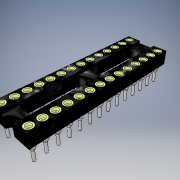
# Autodesk Inventor part: DIL28-Socket
Saved by Autodesk Inventor 2018 (Build 220112000, 112)
## iProperties
Created: 2020-04-18
Part Number: DIL28-Socket
Material: Všeobecné
Document SubType Name: Modeling
Designer: Jozko Mrkvicka
Density: 1 g/cm^3
Appearance: Výchozí
Author: Jozko Mrkvicka
Autodesk Inventor part; units mm, degrees
ref_plane "YZ Plane" through (0, 0, 0) normal (1, 0, 0) x (0, 1, 0)
ref_plane "XZ Plane" through (0, 0, 0) normal (0, 1, 0) x (-1, 0, 0)
ref_plane "XY Plane" through (0, 0, 0) normal (0, 0, 1) x (1, 0, 0)
sketch "Náčrt1" plane through (0, 0, 0) normal (0, 1, 0) x (-1, 0, 0)
  line L0 (10.16, 0) -> (10.16, -35.56)
  line L1 (10.16, -35.56) -> (0, -35.56)
  line L2 (0, -35.56) -> (0, 0)
  line L3 (0, 0) -> (3.175, 0)
  line L4 (3.175, -35.56) -> (0, -35.56)
  line L5 (0, -35.56) -> (0, 0)
  line L6 (10.16, 0) -> (6.985, 0)
  line L7 (6.985, -35.56) -> (10.16, -35.56)
  line L8 (10.16, -35.56) -> (10.16, 0)
  line L9 (3.81, -3.175) -> (6.35, -3.175)
  line L10 (6.985, -35.56) -> (3.175, -35.56)
  line L11 (3.81, -32.385) -> (6.35, -32.385)
  line L12 (3.81, -16.1925) -> (6.35, -16.1925)
  line L13 (6.35, -19.3675) -> (3.81, -19.3675)
  line L14 (6.985, -3.81) -> (6.985, -15.5575)
  line L15 (6.985, -20.0025) -> (6.985, -31.75)
  line L16 (3.175, -3.81) -> (3.175, -15.5575)
  line L17 (3.175, -20.0025) -> (3.175, -31.75)
  arc A0 (3.81, 0) -> (6.35, 0) centre (5.08, 0) ccw
  line L18 (0, 0) -> (3.81, 0)
  line L19 (6.35, 0) -> (10.16, 0)
  line L20 (6.985, 0) -> (6.35, 0)
  line L21 (3.81, 0) -> (3.175, 0)
  arc A1 (6.985, -3.81) -> (6.35, -3.175) centre (6.35, -3.81) ccw
  arc A2 (3.81, -3.175) -> (3.175, -3.81) centre (3.81, -3.81) ccw
  arc A3 (3.175, -15.5575) -> (3.81, -16.1925) centre (3.81, -15.5575) ccw
  arc A4 (6.35, -16.1925) -> (6.985, -15.5575) centre (6.35, -15.5575) ccw
  arc A5 (6.985, -20.0025) -> (6.35, -19.3675) centre (6.35, -20.0025) ccw
  arc A6 (3.81, -19.3675) -> (3.175, -20.0025) centre (3.81, -20.0025) ccw
  arc A7 (6.35, -32.385) -> (6.985, -31.75) centre (6.35, -31.75) ccw
  arc A8 (3.175, -31.75) -> (3.81, -32.385) centre (3.81, -31.75) ccw
  dimension "d0" = 10.16
  dimension "d1" = 35.56
  dimension "d6" = 2.54
  dimension "d7" = 0.635
  constraints: 44 end point, 18 point on circle, 16 tangent, 13 parallel, 9 centre point, 8 horizontal, 7 equal radius, 6 perpendicular, 2 point on line
  measures "d0" distance of L0.end L1.end
  measures "d1" distance of L0.start L0.end
  measures "d6" diameter of A0
  measures "d7" radius of A1
extrude "Vysunutí1" add sketch "Náčrt1" along normal blind 3.175
sketch "Náčrt2" plane through (0, 3.175, 0) normal (0, 1, 0) x (1, 0, 0)
  line L0 (-6.985, 3.81) -> (-6.985, 15.5575) projected
  line L1 (-6.985, 3.81) -> (-3.1004, 3.81)
  line L2 (0, 35.56) -> (-10.16, 35.56) projected
  line L3 (-6.985, 3.81) -> (-3.175, 3.81)
  line L4 (-3.175, 3.81) -> (-3.175, 35.56)
  line L5 (-3.175, 35.56) -> (-6.985, 35.56)
  line L6 (-6.985, 35.56) -> (-6.985, 3.81)
  line L7 (-3.81, 0) -> (0, 0) projected
  line L8 (-6.985, 3.81) -> (-3.175, 3.81)
  line L9 (-3.175, 3.81) -> (-3.175, 0)
  line L10 (-3.175, 0) -> (-6.985, 0)
  line L11 (-6.985, 0) -> (-6.985, 3.81)
  constraints: 18 end point, 4 parallel, 3 horizontal, 2 perpendicular, 2 point on line
extrude "Vysunutí2" cut sketch "Náčrt2" against normal blind 0.635
sketch "Náčrt3" plane through (0, 0, 0) normal (0, -1, 0) x (1, 0, 0)
  circle A0 centre (-1.27, -1.27) radius 0.635
  circle A1 centre (-1.27, -3.81) radius 0.635
  circle A2 centre (-1.27, -6.35) radius 0.635
  circle A3 centre (-1.27, -8.89) radius 0.635
  circle A4 centre (-1.27, -11.43) radius 0.635
  circle A5 centre (-1.27, -13.97) radius 0.635
  circle A6 centre (-1.27, -16.51) radius 0.635
  circle A7 centre (-1.27, -19.05) radius 0.635
  circle A8 centre (-1.27, -21.59) radius 0.635
  circle A9 centre (-8.89, -1.27) radius 0.635
  circle A10 centre (-8.89, -3.81) radius 0.635
  circle A11 centre (-8.89, -6.35) radius 0.635
  circle A12 centre (-8.89, -8.89) radius 0.635
  circle A13 centre (-8.89, -34.29) radius 0.635
  circle A14 centre (-8.89, -31.75) radius 0.635
  circle A15 centre (-8.89, -29.21) radius 0.635
  circle A16 centre (-8.89, -26.67) radius 0.635
  circle A17 centre (-8.89, -24.13) radius 0.635
  circle A18 centre (-8.89, -21.59) radius 0.635
  circle A19 centre (-8.89, -19.05) radius 0.635
  circle A20 centre (-8.89, -16.51) radius 0.635
  circle A21 centre (-8.89, -13.97) radius 0.635
  circle A22 centre (-8.89, -11.43) radius 0.635
  circle A23 centre (-1.27, -34.29) radius 0.635
  circle A24 centre (-1.27, -31.75) radius 0.635
  circle A25 centre (-1.27, -29.21) radius 0.635
  circle A26 centre (-1.27, -26.67) radius 0.635
  circle A27 centre (-1.27, -24.13) radius 0.635
  point P0 (0, 0)
  point P1 (-8.89, -1.27)
  point P2 (-8.89, -3.81)
  point P3 (-8.89, -6.35)
  point P4 (-8.89, -8.89)
  point P5 (-8.89, -11.43)
  point P6 (-8.89, -13.97)
  point P7 (-8.89, -16.51)
  point P8 (-8.89, -19.05)
  point P9 (-8.89, -21.59)
  point P10 (-8.89, -24.13)
  point P11 (-8.89, -26.67)
  point P12 (-8.89, -29.21)
  point P13 (-8.89, -31.75)
  point P14 (-8.89, -34.29)
  point P15 (-1.27, -1.27)
  point P16 (-1.27, -3.81)
  point P17 (-1.27, -11.43)
  point P18 (-1.27, -13.97)
  point P19 (-1.27, -16.51)
  point P20 (-1.27, -19.05)
  point P21 (-1.27, -21.59)
  point P22 (-1.27, -24.13)
  point P23 (-1.27, -26.67)
  point P24 (-1.27, -29.21)
  point P25 (-1.27, -31.75)
  point P26 (-1.27, -34.29)
  constraints: 28 centre point, 1 coincident
extrude "Vysunutí3" add sketch "Náčrt3" along normal blind 1.905
chamfer "Zkosení1" distance 0.3175 distance2 0.635 1 edges at (-1.905, -1.905, -1.27) measured on face at (-1.0935, -1.905, -1.2787)
chamfer "Zkosení2" distance 0.3175 distance2 0.635 1 edges at (-1.905, -1.905, -13.97) measured on face at (-1.4636, -1.905, -14.0177)
chamfer "Zkosení3" distance 0.3175 distance2 0.635 1 edges at (-1.905, -1.905, -3.81) measured on face at (-1.2445, -1.905, -4.0201)
chamfer "Zkosení4" distance 0.3175 distance2 0.635 1 edges at (-9.525, -1.905, -1.27) measured on face at (-8.6964, -1.905, -1.419)
chamfer "Zkosení5" distance 0.3175 distance2 0.635 1 edges at (-9.525, -1.905, -3.81) measured on face at (-8.6964, -1.905, -3.959)
chamfer "Zkosení6" distance 0.3175 distance2 0.635 1 edges at (-9.525, -1.905, -6.35) measured on face at (-8.6964, -1.905, -6.499)
chamfer "Zkosení7" distance 0.3175 distance2 0.635 1 edges at (-9.525, -1.905, -8.89) measured on face at (-8.6783, -1.905, -9.0867)
chamfer "Zkosení8" distance 0.3175 distance2 0.635 1 edges at (-9.525, -1.905, -11.43) measured on face at (-8.6783, -1.905, -11.6267)
chamfer "Zkosení9" distance 0.3175 distance2 0.635 1 edges at (-9.525, -1.905, -13.97) measured on face at (-8.6783, -1.905, -14.1667)
chamfer "Zkosení10" distance 0.3175 distance2 0.635 1 edges at (-1.905, -1.905, -6.35) measured on face at (-1.0645, -1.905, -6.4007)
chamfer "Zkosení11" distance 0.3175 distance2 0.635 1 edges at (-1.905, -1.905, -8.89) measured on face at (-1.4636, -1.905, -8.9377)
chamfer "Zkosení12" distance 0.3175 distance2 0.635 1 edges at (-1.905, -1.905, -11.43) measured on face at (-1.4636, -1.905, -11.4777)
chamfer "Zkosení13" distance 0.3175 distance2 0.635 1 edges at (-1.905, -1.905, -16.51) measured on face at (-1.0826, -1.905, -16.5129)
chamfer "Zkosení14" distance 0.3175 distance2 0.635 1 edges at (-9.525, -1.905, -16.51) measured on face at (-8.7026, -1.905, -16.4116)
chamfer "Zkosení15" distance 0.3175 distance2 0.635 1 edges at (-9.525, -1.905, -19.05) measured on face at (-8.7026, -1.905, -18.9516)
chamfer "Zkosení16" distance 0.3175 distance2 0.635 1 edges at (-1.905, -1.905, -19.05) measured on face at (-1.0826, -1.905, -19.0529)
chamfer "Zkosení17" distance 0.3175 distance2 0.635 1 edges at (-1.905, -1.905, -21.59) measured on face at (-1.0826, -1.905, -21.5929)
chamfer "Zkosení18" distance 0.3175 distance2 0.635 1 edges at (-1.905, -1.905, -24.13) measured on face at (-1.0826, -1.905, -24.1329)
chamfer "Zkosení19" distance 0.3175 distance2 0.635 1 edges at (-1.905, -1.905, -26.67) measured on face at (-1.0826, -1.905, -26.6729)
chamfer "Zkosení20" distance 0.3175 distance2 0.635 1 edges at (-1.905, -1.905, -29.21) measured on face at (-1.0826, -1.905, -29.2129)
chamfer "Zkosení21" distance 0.3175 distance2 0.635 1 edges at (-1.905, -1.905, -31.75) measured on face at (-1.2445, -1.905, -31.9357)
chamfer "Zkosení22" distance 0.3175 distance2 0.635 1 edges at (-1.905, -1.905, -34.29) measured on face at (-1.3451, -1.905, -34.0921)
chamfer "Zkosení23" distance 0.3175 distance2 0.635 1 edges at (-9.525, -1.905, -34.29) measured on face at (-9.2437, -1.905, -34.1259)
chamfer "Zkosení24" distance 0.3175 distance2 0.635 1 edges at (-9.525, -1.905, -31.75) measured on face at (-8.8645, -1.905, -31.9357)
chamfer "Zkosení25" distance 0.3175 distance2 0.635 1 edges at (-9.525, -1.905, -29.21) measured on face at (-8.7026, -1.905, -29.1116)
chamfer "Zkosení26" distance 0.3175 distance2 0.635 1 edges at (-9.525, -1.905, -26.67) measured on face at (-8.7026, -1.905, -26.5716)
chamfer "Zkosení27" distance 0.3175 distance2 0.635 1 edges at (-9.525, -1.905, -24.13) measured on face at (-8.7026, -1.905, -24.0316)
chamfer "Zkosení28" distance 0.3175 distance2 0.635 1 edges at (-9.525, -1.905, -21.59) measured on face at (-8.7026, -1.905, -21.4916)
sketch "Náčrt4" plane through (-1.27, -1.905, -1.27) normal (0, -1, 0) x (1, 0, 0)
  circle A0 centre (0, 0) radius 0.3175 projected
  circle A1 centre (0, 0) radius 0.3175
  circle A2 centre (0, -2.5422) radius 0.3153
  circle A3 centre (0, -5.08) radius 0.3175 projected
  circle A4 centre (0, -5.08) radius 0.3175
  circle A5 centre (0, -7.62) radius 0.3175 projected
  circle A6 centre (0, -7.62) radius 0.3175
  circle A7 centre (0, -10.16) radius 0.3175 projected
  circle A8 centre (0, -10.16) radius 0.3175
  circle A9 centre (0, -12.7) radius 0.3175 projected
  circle A10 centre (0, -12.7) radius 0.3175
  circle A11 centre (0, -15.24) radius 0.3175 projected
  circle A12 centre (0, -15.24) radius 0.3175
  circle A13 centre (0, -17.78) radius 0.3175 projected
  circle A14 centre (0, -17.78) radius 0.3175
  circle A15 centre (0, -20.32) radius 0.3175 projected
  circle A16 centre (0, -20.32) radius 0.3175
  circle A17 centre (0, -22.86) radius 0.3175 projected
  circle A18 centre (0, -22.86) radius 0.3175
  circle A19 centre (0, -25.4) radius 0.3175
  circle A20 centre (0, -27.94) radius 0.3175 projected
  circle A21 centre (0, -27.94) radius 0.3175
  circle A22 centre (0, -30.48) radius 0.3175
  circle A23 centre (0, -33.02) radius 0.3175 projected
  circle A24 centre (0, -33.02) radius 0.3175
  circle A25 centre (-7.62, -33.02) radius 0.3175 projected
  circle A26 centre (-7.62, -33.02) radius 0.3175
  circle A27 centre (-7.62, -30.48) radius 0.3175
  circle A28 centre (-7.62, -27.94) radius 0.3175
  circle A29 centre (-7.62, -25.4) radius 0.3175 projected
  circle A30 centre (-7.62, -25.4) radius 0.3175
  circle A31 centre (-7.62, -22.86) radius 0.3175 projected
  circle A32 centre (-7.62, -22.86) radius 0.3175
  circle A33 centre (-7.62, -20.32) radius 0.3175
  circle A34 centre (-7.62, -17.78) radius 0.3175 projected
  circle A35 centre (-7.62, -17.78) radius 0.3175
  circle A36 centre (-7.62, -15.24) radius 0.3175 projected
  circle A37 centre (-7.62, -15.24) radius 0.3175
  circle A38 centre (-7.62, -12.7) radius 0.3175
  circle A39 centre (-7.62, -10.16) radius 0.3175 projected
  circle A40 centre (-7.62, -10.16) radius 0.3175
  circle A41 centre (-7.62, -7.62) radius 0.3175
  circle A42 centre (-7.62, -5.08) radius 0.3175
  circle A43 centre (-7.62, -2.54) radius 0.3175
  circle A44 centre (-7.62, 0) radius 0.3175
  point P0 (1.27, 1.27)
  constraints: 28 centre point, 23 coincident
extrude "Vysunutí4" add sketch "Náčrt4" along normal blind 2.54
fillet "Zaoblení1" radius 0.127 28 edges at (-9.2075, -4.445, -1.27) (-9.2075, -4.445, -3.81) (-9.2075, -4.445, -6.35) (-1.5875, -4.445, -1.27) (-1.5853, -4.445, -3.8122) (-1.5875, -4.445, -6.35) (-9.2075, -4.445, -8.89) (-9.2075, -4.445, -11.43) (-9.2075, -4.445, -13.97) (-9.2075, -4.445, -16.51) (-9.2075, -4.445, -19.05) (-9.2075, -4.445, -21.59) (-9.2075, -4.445, -24.13) (-9.2075, -4.445, -26.67) (-9.2075, -4.445, -29.21) (-9.2075, -4.445, -31.75) (-9.2075, -4.445, -34.29) (-1.5875, -4.445, -34.29) (-1.5875, -4.445, -31.75) (-1.5875, -4.445, -29.21) (-1.5875, -4.445, -26.67) (-1.5875, -4.445, -24.13) (-1.5875, -4.445, -21.59) (-1.5875, -4.445, -19.05) (-1.5875, -4.445, -16.51) (-1.5875, -4.445, -13.97) (-1.5875, -4.445, -11.43) (-1.5875, -4.445, -8.89)
sketch "Náčrt5" plane through (0, 3.175, 0) normal (0, 1, 0) x (1, 0, 0)
  circle A0 centre (-1.27, 1.27) radius 0.635 projected
  circle A1 centre (-1.27, 26.67) radius 0.635 projected
  circle A2 centre (-1.27, 31.75) radius 0.635 projected
  circle A3 centre (-8.89, 11.43) radius 0.635 projected
  circle A4 centre (-8.89, 16.51) radius 0.635 projected
  circle A5 centre (-8.89, 21.59) radius 0.635 projected
  circle A6 centre (-8.89, 26.67) radius 0.635 projected
  circle A7 centre (-8.89, 31.75) radius 0.635 projected
  circle A8 centre (-8.89, 8.89) radius 0.635 projected
  circle A9 centre (-8.89, 3.81) radius 0.635 projected
  circle A10 centre (-1.27, 21.59) radius 0.635 projected
  circle A11 centre (-1.27, 16.51) radius 0.635 projected
  circle A12 centre (-1.27, 11.43) radius 0.635 projected
  circle A13 centre (-1.27, 6.35) radius 0.635 projected
  circle A14 centre (-1.27, 1.27) radius 0.635 projected
  circle A15 centre (-1.27, 3.81) radius 0.635 projected
  circle A16 centre (-1.27, 8.89) radius 0.635 projected
  circle A17 centre (-1.27, 13.97) radius 0.635 projected
  circle A18 centre (-1.27, 19.05) radius 0.635 projected
  circle A19 centre (-8.89, 1.27) radius 0.635 projected
  circle A20 centre (-8.89, 6.35) radius 0.635 projected
  circle A21 centre (-8.89, 34.29) radius 0.635 projected
  circle A22 centre (-8.89, 29.21) radius 0.635 projected
  circle A23 centre (-8.89, 24.13) radius 0.635 projected
  circle A24 centre (-8.89, 19.05) radius 0.635 projected
  circle A25 centre (-8.89, 13.97) radius 0.635 projected
  circle A26 centre (-1.27, 34.29) radius 0.635 projected
  circle A27 centre (-1.27, 29.21) radius 0.635 projected
  circle A28 centre (-1.27, 24.13) radius 0.635 projected
  arc A29 (-6.35, 32.385) -> (-6.985, 31.75) centre (-6.35, 31.75) ccw projected
  line L0 (-6.985, 31.75) -> (-6.985, 20.0025) projected
  arc A30 (-6.985, 20.0025) -> (-6.35, 19.3675) centre (-6.35, 20.0025) ccw projected
  line L1 (-6.35, 19.3675) -> (-3.81, 19.3675) projected
  arc A31 (-3.81, 19.3675) -> (-3.175, 20.0025) centre (-3.81, 20.0025) ccw projected
  line L2 (-3.175, 20.0025) -> (-3.175, 31.75) projected
  arc A32 (-3.175, 31.75) -> (-3.81, 32.385) centre (-3.81, 31.75) ccw projected
  line L3 (-3.81, 32.385) -> (-6.35, 32.385) projected
  arc A33 (-6.35, 16.1925) -> (-6.985, 15.5575) centre (-6.35, 15.5575) ccw projected
  line L4 (-6.985, 15.5575) -> (-6.985, 3.81) projected
  arc A34 (-6.985, 3.81) -> (-6.35, 3.175) centre (-6.35, 3.81) ccw projected
  line L5 (-6.35, 3.175) -> (-3.81, 3.175) projected
  arc A35 (-3.81, 3.175) -> (-3.175, 3.81) centre (-3.81, 3.81) ccw projected
  line L6 (-3.175, 3.81) -> (-3.175, 15.5575) projected
  arc A36 (-3.175, 15.5575) -> (-3.81, 16.1925) centre (-3.81, 15.5575) ccw projected
  line L7 (-3.81, 16.1925) -> (-6.35, 16.1925) projected
  line L8 (0, 0) -> (0, 35.56) projected
  line L9 (-3.81, 0) -> (0, 0) projected
  arc A37 (-3.81, 0) -> (-6.35, 0) centre (-5.08, 0) ccw projected
  line L10 (-10.16, 0) -> (-6.35, 0) projected
  line L11 (-10.16, 35.56) -> (-10.16, 0) projected
  line L12 (0, 35.56) -> (-10.16, 35.56) projected
extrude "Vysunutí5" cut sketch "Náčrt5" against normal blind 0.635 contours A0 | A1 | A2 | A3 | A4 | A5 | A6 | A7 | A8 | A9 | A10 | A11 | A12 | A13 | A15 | A16 | A17 | A18 | A19 | A20 | A21 | A22 | A23 | A24 | A25 | A26 | A27 | A28
sketch "Náčrt6" plane through (-1.27, 2.54, -1.27) normal (0, 1, 0) x (1, 0, 0)
  circle A0 centre (-7.62, 0) radius 0.3175 projected
  circle A1 centre (-7.62, 2.54) radius 0.3175 projected
  circle A2 centre (-7.62, 5.08) radius 0.3175 projected
  circle A3 centre (-7.62, 7.62) radius 0.3175 projected
  circle A4 centre (-7.62, 10.16) radius 0.3175 projected
  circle A5 centre (-7.62, 12.7) radius 0.3175 projected
  circle A6 centre (-7.62, 15.24) radius 0.3175 projected
  circle A7 centre (-7.62, 17.78) radius 0.3175 projected
  circle A8 centre (-7.62, 20.32) radius 0.3175 projected
  circle A9 centre (-7.62, 22.86) radius 0.3175 projected
  circle A10 centre (-7.62, 25.4) radius 0.3175 projected
  circle A11 centre (-7.62, 27.94) radius 0.3175 projected
  circle A12 centre (-7.62, 30.48) radius 0.3175 projected
  circle A13 centre (-7.62, 33.02) radius 0.3175 projected
  circle A14 centre (0, 33.02) radius 0.3175 projected
  circle A15 centre (0, 30.48) radius 0.3175 projected
  circle A16 centre (0, 27.94) radius 0.3175 projected
  circle A17 centre (0, 25.4) radius 0.3175 projected
  circle A18 centre (0, 22.86) radius 0.3175 projected
  circle A19 centre (0, 20.32) radius 0.3175 projected
  circle A20 centre (0, 17.78) radius 0.3175 projected
  circle A21 centre (0, 15.24) radius 0.3175 projected
  circle A22 centre (0, 12.7) radius 0.3175 projected
  circle A23 centre (0, 10.16) radius 0.3175 projected
  circle A24 centre (0, 7.62) radius 0.3175 projected
  circle A25 centre (0, 5.08) radius 0.3175 projected
  circle A26 centre (0, 2.54) radius 0.3175 projected
  circle A27 centre (0, 0) radius 0.3175 projected
  point P0 (1.27, -1.27)
  point P1 (0, 2.8575)
  constraints: 1 vertical alignment
extrude "Vysunutí6" cut sketch "Náčrt6" against normal blind 1.27
sketch "Náčrt7" plane through (0, 3.175, 0) normal (0, 1, 0) x (1, 0, 0)
  circle A0 centre (-8.89, 1.27) radius 0.9525
  circle A1 centre (-8.89, 8.89) radius 0.9525
  circle A2 centre (-8.89, 3.81) radius 0.9525
  circle A3 centre (-8.89, 6.35) radius 0.9525
  circle A4 centre (-8.89, 11.43) radius 0.9525
  circle A5 centre (-8.89, 13.97) radius 0.9525
  circle A6 centre (-8.89, 16.51) radius 0.9525
  circle A7 centre (-8.89, 19.05) radius 0.9525
  circle A8 centre (-8.89, 21.59) radius 0.9525
  circle A9 centre (-8.89, 24.13) radius 0.9525
  circle A10 centre (-8.89, 26.67) radius 0.9525
  circle A11 centre (-8.89, 29.21) radius 0.9525
  circle A12 centre (-8.89, 31.75) radius 0.9525
  circle A13 centre (-8.89, 34.29) radius 0.9525
  circle A14 centre (-1.27, 1.27) radius 0.9525
  circle A15 centre (-1.27, 3.81) radius 0.9525
  circle A16 centre (-1.27, 6.35) radius 0.9525
  circle A17 centre (-1.27, 8.89) radius 0.9525
  circle A18 centre (-1.27, 11.43) radius 0.9525
  circle A19 centre (-1.27, 13.97) radius 0.9525
  circle A20 centre (-1.27, 16.51) radius 0.9525
  circle A21 centre (-1.27, 19.05) radius 0.9525
  circle A22 centre (-1.27, 21.59) radius 0.9525
  circle A23 centre (-1.27, 24.13) radius 0.9525
  circle A24 centre (-1.27, 26.67) radius 0.9525
  circle A25 centre (-1.27, 29.21) radius 0.9525
  circle A26 centre (-1.27, 31.75) radius 0.9525
  circle A27 centre (-1.27, 34.29) radius 0.9525
  circle A28 centre (-1.27, 1.27) radius 0.635 projected
  circle A29 centre (-1.27, 3.81) radius 0.3175 projected
  circle A30 centre (-1.27, 6.35) radius 0.3175 projected
  circle A31 centre (-1.27, 8.89) radius 0.3175 projected
  circle A32 centre (-1.27, 11.43) radius 0.3175 projected
  circle A33 centre (-1.27, 13.97) radius 0.3175 projected
  circle A34 centre (-1.27, 16.51) radius 0.635 projected
  circle A35 centre (-1.27, 21.59) radius 0.3175 projected
  circle A36 centre (-1.27, 24.13) radius 0.3175 projected
  circle A37 centre (-1.27, 26.67) radius 0.3175 projected
  circle A38 centre (-1.27, 29.21) radius 0.3175 projected
  circle A39 centre (-1.27, 31.75) radius 0.635 projected
  circle A40 centre (-1.27, 34.29) radius 0.3175 projected
  circle A41 centre (-8.89, 34.29) radius 0.3175 projected
  circle A42 centre (-8.89, 31.75) radius 0.3175 projected
  circle A43 centre (-8.89, 29.21) radius 0.3175 projected
  circle A44 centre (-8.89, 26.67) radius 0.3175 projected
  circle A45 centre (-8.89, 24.13) radius 0.3175 projected
  circle A46 centre (-8.89, 21.59) radius 0.3175 projected
  circle A47 centre (-8.89, 19.05) radius 0.3175 projected
  circle A48 centre (-8.89, 16.51) radius 0.3175 projected
  circle A49 centre (-8.89, 13.97) radius 0.3175 projected
  circle A50 centre (-8.89, 11.43) radius 0.3175 projected
  circle A51 centre (-8.89, 8.89) radius 0.3175 projected
  circle A52 centre (-8.89, 6.35) radius 0.3175 projected
  circle A53 centre (-8.89, 3.81) radius 0.3175 projected
  circle A54 centre (-8.89, 1.27) radius 0.635 projected
  circle A55 centre (-8.89, 3.81) radius 0.635 projected
  circle A56 centre (-8.89, 6.35) radius 0.635 projected
  circle A57 centre (-1.27, 26.67) radius 0.635 projected
  circle A58 centre (-1.27, 31.75) radius 0.635 projected
  circle A59 centre (-8.89, 11.43) radius 0.635 projected
  circle A60 centre (-8.89, 16.51) radius 0.635 projected
  circle A61 centre (-8.89, 21.59) radius 0.635 projected
  circle A62 centre (-8.89, 26.67) radius 0.635 projected
  circle A63 centre (-8.89, 31.75) radius 0.635 projected
  circle A64 centre (-8.89, 8.89) radius 0.635 projected
  circle A65 centre (-8.89, 3.81) radius 0.635 projected
  circle A66 centre (-1.27, 21.59) radius 0.635 projected
  circle A67 centre (-1.27, 16.51) radius 0.635 projected
  circle A68 centre (-1.27, 11.43) radius 0.635 projected
  circle A69 centre (-1.27, 6.35) radius 0.635 projected
  circle A70 centre (-1.27, 1.27) radius 0.635 projected
  circle A71 centre (-1.27, 3.81) radius 0.635 projected
  circle A72 centre (-1.27, 8.89) radius 0.635 projected
  circle A73 centre (-1.27, 13.97) radius 0.635 projected
  circle A74 centre (-1.27, 19.05) radius 0.635 projected
  circle A75 centre (-8.89, 1.27) radius 0.635 projected
  circle A76 centre (-8.89, 6.35) radius 0.635 projected
  circle A77 centre (-8.89, 34.29) radius 0.635 projected
  circle A78 centre (-8.89, 29.21) radius 0.635 projected
  circle A79 centre (-8.89, 24.13) radius 0.635 projected
  circle A80 centre (-8.89, 19.05) radius 0.635 projected
  circle A81 centre (-8.89, 13.97) radius 0.635 projected
  circle A82 centre (-1.27, 34.29) radius 0.635 projected
  circle A83 centre (-1.27, 29.21) radius 0.635 projected
  circle A84 centre (-1.27, 24.13) radius 0.635 projected
  arc A85 (-6.35, 32.385) -> (-6.985, 31.75) centre (-6.35, 31.75) ccw projected
  line L0 (-6.985, 31.75) -> (-6.985, 20.0025) projected
  arc A86 (-6.985, 20.0025) -> (-6.35, 19.3675) centre (-6.35, 20.0025) ccw projected
  line L1 (-6.35, 19.3675) -> (-3.81, 19.3675) projected
  arc A87 (-3.81, 19.3675) -> (-3.175, 20.0025) centre (-3.81, 20.0025) ccw projected
  line L2 (-3.175, 20.0025) -> (-3.175, 31.75) projected
  arc A88 (-3.175, 31.75) -> (-3.81, 32.385) centre (-3.81, 31.75) ccw projected
  line L3 (-3.81, 32.385) -> (-6.35, 32.385) projected
  arc A89 (-6.35, 16.1925) -> (-6.985, 15.5575) centre (-6.35, 15.5575) ccw projected
  line L4 (-6.985, 15.5575) -> (-6.985, 3.81) projected
  arc A90 (-6.985, 3.81) -> (-6.35, 3.175) centre (-6.35, 3.81) ccw projected
  line L5 (-6.35, 3.175) -> (-3.81, 3.175) projected
  arc A91 (-3.81, 3.175) -> (-3.175, 3.81) centre (-3.81, 3.81) ccw projected
  line L6 (-3.175, 3.81) -> (-3.175, 15.5575) projected
  arc A92 (-3.175, 15.5575) -> (-3.81, 16.1925) centre (-3.81, 15.5575) ccw projected
  line L7 (-3.81, 16.1925) -> (-6.35, 16.1925) projected
  line L8 (0, 0) -> (0, 35.56) projected
  line L9 (-3.81, 0) -> (0, 0) projected
  arc A93 (-3.81, 0) -> (-6.35, 0) centre (-5.08, 0) ccw projected
  line L10 (-10.16, 0) -> (-6.35, 0) projected
  line L11 (-10.16, 35.56) -> (-10.16, 0) projected
  line L12 (0, 35.56) -> (-10.16, 35.56) projected
  circle A94 centre (-8.89, 3.81) radius 0.635 projected
  constraints: 28 centre point, 26 coincident
extrude "Vysunutí7" cut sketch "Náčrt7" against normal blind 0.0254 contours A0 | A1 | A2 | A3 | A4 | A5 | A6 | A7 | A8 | A9 | A10 | A11 | A12 | A13 | A14 | A15 | A16 | A17 | A18 | A19 | A20 | A21 | A22 | A23 | A24 | A25 | A26 | A27
